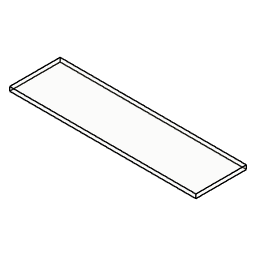
Initial Design Idea (Autodesk Fusion 360 archive; units mm, degrees)
design "Front-Back"
Autodesk Fusion 360 part; units mm, degrees
sketch "Sketch1" plane through (0, 0, 0) normal (0, 0, 1) x (1, 0, 0)
  line L0 (115.3, 31.25) -> (-115.3, 31.25)
  line L1 (-115.3, 31.25) -> (-115.3, -31.25)
  line L2 (-115.3, -31.25) -> (115.3, -31.25)
  line L3 (115.3, -31.25) -> (115.3, 31.25)
  line L4 (115.3, 31.25) -> (-115.3, -31.25) construction
  line L5 (-115.3, 31.25) -> (115.3, -31.25) construction
  dimension "d1" = 230.6
  dimension "d2" = 62.5
  constraint horizontal L0
  constraint perpendicular L0 L1
  constraint parallel L0 L2
  constraint parallel L1 L3
  constraint coincident L4 origin
  constraint coincident L5 origin
  measures "d1" distance of L0.start L0.end
  measures "d2" distance of L0.end L1.end
extrude "Extrude1" add sketch "Sketch1" along normal blind 5

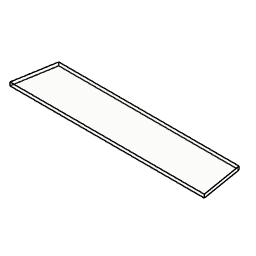
design "Side Panels"
Autodesk Fusion 360 part; units mm, degrees
sketch "Sketch1" plane through (0, 0, 0) normal (0, 0, 1) x (1, 0, 0)
  line L0 (135, -31.25) -> (-135, -31.25)
  line L1 (-135, -31.25) -> (-135, 31.25)
  line L2 (-135, 31.25) -> (135, 31.25)
  line L3 (135, 31.25) -> (135, -31.25)
  line L4 (135, -31.25) -> (-135, 31.25) construction
  line L5 (-135, -31.25) -> (135, 31.25) construction
  line L6 (-135, -31.25) -> (-145.5, -31.25)
  line L7 (-135, 31.25) -> (-145.5, -31.25)
  line L8 (135, -31.25) -> (145.5, -31.25)
  line L9 (135, 31.25) -> (145.5, -31.25)
  dimension "d1" = 62.5
  dimension "d2" = 270
  dimension "d5" = 10.5
  dimension "d6" = 10.5
  constraint horizontal L0
  constraint perpendicular L0 L1
  constraint parallel L0 L2
  constraint parallel L1 L3
  constraint coincident L4 origin
  constraint coincident L5 origin
  constraint perpendicular L1 L6
  constraint perpendicular L3 L8
  measures "d1" distance of L0.end L1.end
  measures "d2" distance of L1.end L2.end
  measures "d5" distance of L0.end L6.end
  measures "d6" distance of L0.start L8.end
extrude "Extrude1" add sketch "Sketch1" along normal blind 5

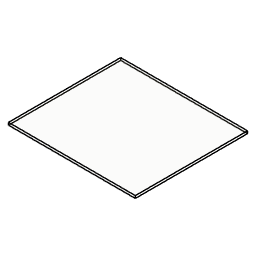
design "Top Cover"
Autodesk Fusion 360 part; units mm, degrees
sketch "Sketch1" plane through (0, 0, 0) normal (0, 0, 1) x (1, 0, 0)
  line L0 (130, -115) -> (-130, -115)
  line L1 (-130, -115) -> (-130, 115)
  line L2 (-130, 115) -> (130, 115)
  line L3 (130, 115) -> (130, -115)
  line L4 (130, -115) -> (-130, 115) construction
  line L5 (-130, -115) -> (130, 115) construction
  dimension "d1" = 260
  dimension "d2" = 230
  constraint horizontal L0
  constraint perpendicular L0 L1
  constraint parallel L0 L2
  constraint parallel L1 L3
  constraint coincident L4 origin
  constraint coincident L5 origin
  measures "d1" distance of L1.end L2.end
  measures "d2" distance of L0.end L1.end
extrude "Extrude1" add sketch "Sketch1" along normal blind 5
